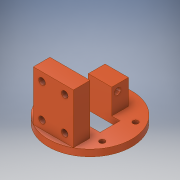
# Autodesk Inventor part: 000.402 - Держатель стержжня
Saved by Autodesk Inventor 2019 (Build 230136000, 136)
## iProperties
Created: 2020-03-21
Part Number: 000.402 - Держатель стержжня
Material: Пластик АБС
Document SubType Name: Modeling
Designer: Петров Иван
Density: 1.06 g/cm^3
Appearance: Гладкий — светло-оранжевый
Author: Петров Иван
Autodesk Inventor part; units mm, degrees
ref_plane "YZ Plane" through (0, 0, 0) normal (1, 0, 0) x (0, 1, 0)
sketch "Эскиз1" plane through (0, 0, 0) normal (0, 1, 0) x (-1, 0, 0)
  circle A0 centre (0, 0) radius 5
  line L0 (0, 0) -> (0, -20)
  circle A1 centre (0, 0) radius 25
  circle A2 centre (0, -20) radius 1.6
  dimension "d0" = 10
  dimension "d1" = 20
  dimension "d2" = 50
  dimension "d3" = 3.2
  constraints: 3 centre point, 3 coincident, 2 end point, 1 vertical
  measures "d0" diameter of A0
  measures "d1" distance of L0.start L0.end
  measures "d2" diameter of A1
  measures "d3" diameter of A2
extrude "Выдавливание1" add sketch "Эскиз1" along normal blind 4 contours A0 | A2 | A1
sketch "Эскиз2" plane through (0, 4, 0) normal (0, 1, 0) x (1, 0, 0)
  line L0 (0, 0) -> (0, 20)
  circle A0 centre (0, 20) radius 1.6
  dimension "d6" = 20
  dimension "d7" = 3.2
  constraints: 2 end point, 1 centre point, 1 coincident, 1 vertical
  measures "d6" distance of L0.start L0.end
  measures "d7" diameter of A0
extrude "Выдавливание2" cut sketch "Эскиз2" against normal blind 8.5
pattern_circular "Круговой массив1" count 6 over 360 about axis through (0, 0, 0) along (0, 1, 0) of "Выдавливание2"
sketch "Эскиз6" plane through (0, 4, 0) normal (0, 1, 0) x (1, 0, 0)
  line L0 (12, -6) -> (12, 6)
  line L1 (12, 6) -> (-12, 6)
  line L2 (-12, 6) -> (-12, -6)
  line L3 (-3, -12) -> (3, -12)
  line L4 (3, -12) -> (3, -6)
  line L5 (-3, -6) -> (-3, -12)
  line L6 (-12, -6) -> (-3, -6)
  line L7 (3, -6) -> (12, -6)
  point P0 (0, 0)
  constraints: 16 end point, 4 parallel, 3 horizontal, 3 perpendicular
extrude "Выдавливание5" cut sketch "Эскиз6" against normal blind 8.5
sketch "Эскиз7" plane through (0, 4, 0) normal (0, 1, 0) x (1, 0, 0)
  line L0 (-12, -6) -> (-12, 6) construction
  line L1 (-12, -6) -> (-12, -12) construction
  line L2 (3, -12) -> (-3, -12) construction
  line L3 (-12, -12) -> (-3, -12) construction
  circle A0 centre (0, 0) radius 25 construction
  line L4 (-12, -12) -> (12, -12)
  line L5 (12, -12) -> (12, -21.9317)
  line L6 (12, -21.9317) -> (-12, -21.9317)
  line L7 (-12, -21.9317) -> (-12, -12)
  dimension "d32" = 24
  constraints: 12 end point, 2 parallel, 1 collinear, 1 horizontal, 1 perpendicular, 1 vertical, 2 other
  measures "d32" distance of L5.end L6.end
extrude "Выдавливание6" add sketch "Эскиз7" along normal blind 30
sketch "Эскиз8" plane through (3, 0, 12) normal (0, 0, -1) x (-1, 0, 0)
  line L0 (3, 0) -> (3, 34)
  line L1 (-9, 34) -> (15, 34) projected
  line L2 (6, 4) -> (6, 0) projected
  line L3 (6, 4) -> (6, 34)
  line L4 (0, 4) -> (-9, 4) projected
  line L5 (0, 4) -> (0, 34)
  line L6 (0, 29) -> (-3.8, 29)
  circle A0 centre (-3.8, 29) radius 2
  dimension "d35" = 3.8
  dimension "d36" = 5
  dimension "d37" = 4
  constraints: 8 end point, 2 perpendicular, 2 point on line, 1 centre point, 1 coincident, 1 midpoint, 1 vertical
  measures "d35" distance of L6.start L6.end
  measures "d36" distance between parallel lines of L1 L6
  measures "d37" diameter of A0
extrude "Выдавливание7" cut sketch "Эскиз8" against normal blind 26.25
ref_plane "РабПлоскость1" through (0, 34, 12) normal (1, 0, 0) x (0, 0, -1)
ref_plane "РабПлоскость2" through (12, 19, 12) normal (0, 1, 0) x (1, 0, 0)
mirror "Зеркальное отражение1" about plane through (12, 19, 12) normal (0, 1, 0) of "Выдавливание7"
mirror "Зеркальное отражение2" about plane through (0, 34, 12) normal (1, 0, 0) of "Выдавливание7", "Зеркальное отражение1"
sketch "Эскиз9" plane through (0, 4, 0) normal (0, 1, 0) x (1, 0, 0)
  line L0 (12, 6) -> (-12, 6) projected
  line L1 (0, 6) -> (0, 16)
  line L2 (0, 16) -> (7, 16)
  line L3 (7, 16) -> (7, 6)
  line L4 (12, 6) -> (12, -6) projected
  point P0 (0, 0)
  dimension "d40" = 10
  dimension "d41" = 5
  constraints: 6 end point, 1 horizontal, 1 midpoint, 1 perpendicular, 1 point on line, 1 vertical
  measures "d40" distance of L1.start L1.end
  measures "d41" distance between parallel lines of L3 L4
extrude "Выдавливание8" add sketch "Эскиз9" along normal blind 15
mirror "Зеркальное отражение3" about plane through (0, 0, 0) normal (1, 0, 0) of "Выдавливание8"
sketch "Эскиз10" plane through (7, 4, -6) normal (1, 0, 0) x (0, 0, -1)
  line L0 (3.5, 15) -> (3.5, 11)
  line L1 (10, 0) -> (10, 15) projected
  circle A0 centre (3.5, 11) radius 2
  point P0 (-6, -4)
  dimension "d44" = 4
  dimension "d45" = 6.5
  dimension "d46" = 4
  constraints: 2 end point, 1 centre point, 1 coincident, 1 vertical
  measures "d44" distance of L0.start L0.end
  measures "d45" distance between parallel lines of L1 L0
  measures "d46" diameter of A0
extrude "Выдавливание9" cut sketch "Эскиз10" against normal blind 53.75
